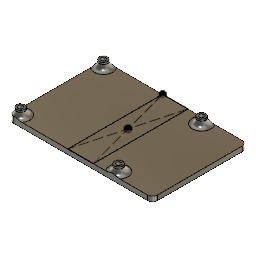
Raspberry Pi mounting (Autodesk Fusion 360 design; units mm, degrees)
Autodesk Fusion 360 part; units mm, degrees
sketch "スケッチ1" plane through (0, 0, 0) normal (0, 0, 1) x (1, 0, 0)
  line L0 (39.5, 28) -> (-39.5, 28)
  line L1 (-42.5, 25) -> (-42.5, -25)
  line L2 (-39.5, -28) -> (39.5, -28)
  line L3 (42.5, -25) -> (42.5, 25)
  line L4 (42.5, 28) -> (-42.5, -28) construction
  line L5 (-42.5, 28) -> (42.5, -28) construction
  arc A0 (-39.5, 28) -> (-42.5, 25) centre (-39.5, 25) ccw
  arc A1 (-42.5, -25) -> (-39.5, -28) centre (-39.5, -25) ccw
  arc A2 (39.5, -28) -> (42.5, -25) centre (39.5, -25) ccw
  arc A3 (42.5, 25) -> (39.5, 28) centre (39.5, 25) ccw
  dimension "d1" = 85
  dimension "d2" = 56
  dimension "d3" = 3
  dimension "d4" = 3
  dimension "d5" = 3
  dimension "d6" = 3
  constraint perpendicular L0 L1
  constraint parallel L0 L2
  constraint parallel L1 L3
  constraint horizontal L0
  constraint coincident L4 origin
  constraint coincident L5 origin
  constraint coincident L5.start L0
  constraint coincident L5.start L1
  constraint tangent L0 A0
  constraint tangent L1 A0
  constraint coincident L4.end L1
  constraint coincident L4.end L2
  constraint tangent L1 A1
  constraint tangent L2 A1
  constraint coincident L5.end L2
  constraint coincident L5.end L3
  constraint tangent L2 A2
  constraint tangent L3 A2
  constraint tangent L3 A3
  constraint tangent L0 A3
  measures "d1" distance of L4.end L5.end
  measures "d2" distance of L5.start L4.end
  measures "d3" radius of A0
  measures "d4" radius of A1
  measures "d5" radius of A2
  measures "d6" radius of A3
extrude "押し出し1" add sketch "スケッチ1" along normal blind 3
sketch "スケッチ2" plane through (0, 0, 3) normal (0, 0, 1) x (-1, 0, 0)
  arc A0 (-42.5, -25) -> (-39.5, -28) centre (-39.5, -25) ccw
  line L0 (-39.5, -28) -> (39.5, -28)
  arc A1 (39.5, -28) -> (42.5, -25) centre (39.5, -25) ccw
  line L1 (42.5, -25) -> (42.5, 25)
  arc A2 (42.5, 25) -> (39.5, 28) centre (39.5, 25) ccw
  line L2 (39.5, 28) -> (-39.5, 28)
  arc A3 (-39.5, 28) -> (-42.5, 25) centre (-39.5, 25) ccw
  line L3 (-42.5, 25) -> (-42.5, -25)
  circle A4 centre (39, 24.5) radius 2.5
  circle A5 centre (-19, 24.5) radius 2.5
  circle A6 centre (39, -24.5) radius 2.5
  circle A7 centre (-19, -24.5) radius 2.5
  dimension "d9" = 5
  dimension "d10" = 3.5
  dimension "d11" = 3.5
  dimension "d14" = -58
  dimension "d15" = -49
  measures "d9" diameter of A4
  measures "d10" distance of L1 A4.centre
  measures "d11" distance of L2 A4.centre
extrude "押し出し2" add sketch "スケッチ2" along normal blind 4 contours A4 | A5 | A6 | A7
fillet "フィレット1" radius 3 4 edges at (-36.6692, -25.404, 3) (-36.6692, 23.596, 3) (21.3308, 23.596, 3) (21.3308, -25.404, 3)
sketch "スケッチ3" plane through (0, 0, 7) normal (0, 0, 1) x (-1, 0, 0)
  circle A0 centre (39, 24.5) radius 1.4
  circle A1 centre (-19, 24.5) radius 1.4
  circle A2 centre (39, -24.5) radius 1.4
  circle A3 centre (-19, -24.5) radius 1.4
  circle A4 centre (39, 24.5) radius 2.5
  dimension "d19" = 2.8
  dimension "d22" = -58
  dimension "d23" = -49
  measures "d19" diameter of A0
extrude "押し出し3" cut sketch "スケッチ3" against normal blind 5 contours A0 | A1 | A2 | A3
sketch "スケッチ4" plane through (0, 0, 3) normal (0, 0, 1) x (-1, 0, 0)
  arc A0 (-23.2426, 28) -> (-14.7574, 28) centre (-19, 24.5) ccw
  line L0 (-23.2426, 28) -> (-39.5, 28)
  arc A1 (-39.5, 28) -> (-42.5, 25) centre (-39.5, 25) ccw
  line L1 (-42.5, 25) -> (-42.5, -25)
  arc A2 (-42.5, -25) -> (-39.5, -28) centre (-39.5, -25) ccw
  line L2 (-39.5, -28) -> (-23.2426, -28)
  arc A3 (-14.7574, -28) -> (-23.2426, -28) centre (-19, -24.5) ccw
  line L3 (-14.7574, -28) -> (34.7574, -28)
  arc A4 (42.5, -20.2574) -> (34.7574, -28) centre (39, -24.5) ccw
  line L4 (42.5, -20.2574) -> (42.5, 20.2574)
  arc A5 (34.7574, 28) -> (42.5, 20.2574) centre (39, 24.5) ccw
  line L5 (34.7574, 28) -> (-14.7574, 28)
  line L6 (7.5, -28) -> (-7.5, -28)
  line L7 (-7.5, -28) -> (-7.5, 28)
  line L8 (-7.5, 28) -> (7.5, 28)
  line L9 (7.5, 28) -> (7.5, -28)
  line L10 (7.5, -28) -> (-7.5, 28) construction
  line L11 (-7.5, -28) -> (7.5, 28) construction
  dimension "d26" = 15
  constraint perpendicular L6 L7
  constraint parallel L6 L8
  constraint parallel L7 L9
  constraint horizontal L6
  constraint coincident L3 L6.start
  constraint coincident L10 origin
  constraint coincident L11 origin
  measures "d26" distance of L7.end L8.end
extrude "押し出し4" [suppressed]
fillet "フィレット2" [suppressed]
sketch "スケッチ5" plane through (0, 0, 3) normal (0, 0, 1) x (-1, 0, 0)
  line L0 (7.5, -27) -> (34.101, -27)
  arc A0 (41.5, -19.601) -> (34.101, -27) centre (39, -24.5) ccw
  line L1 (41.5, -19.601) -> (41.5, 19.601)
  arc A1 (34.101, 27) -> (41.5, 19.601) centre (39, 24.5) ccw
  line L2 (34.101, 27) -> (7.5, 27)
  line L3 (7.5, 27) -> (7.5, -27)
  line L4 (-39.0074, 21.5124) -> (-39.0074, -21.6595) construction
  line L5 (-39.0074, -21.6595) -> (-27.0074, -21.6595) construction
  line L6 (-27.0074, -21.6595) -> (-27.0074, 21.5124) construction
  line L7 (-27.0074, 21.5124) -> (-39.0074, 21.5124) construction
  constraint perpendicular L4 L5
  constraint parallel L4 L6
  constraint parallel L5 L7
extrude "押し出し6" [suppressed]
